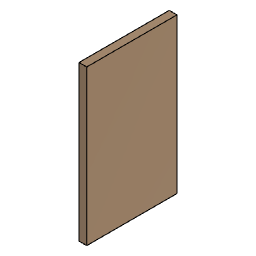
Connection box side panel (Autodesk Fusion 360 design; units mm, degrees)
Autodesk Fusion 360 part; units mm, degrees
sketch "Sketch1" plane through (0, 0, 0) normal (1, 0, 0) x (0, 1, 0)
  line L0 (35, 60) -> (-35, 60)
  line L1 (-35, 60) -> (-35, -60)
  line L2 (-35, -60) -> (35, -60)
  line L3 (35, -60) -> (35, 60)
  line L4 (35, 60) -> (-35, -60) construction
  line L5 (-35, 60) -> (35, -60) construction
  dimension "d1" = 70
  dimension "d2" = 120
  constraint perpendicular L0 L1
  constraint parallel L0 L2
  constraint parallel L1 L3
  constraint horizontal L0
  constraint coincident L4 origin
  constraint coincident L5 origin
  measures "d1" distance of L1.end L2.end
  measures "d2" distance of L0.end L1.end
extrude "Extrude1" add sketch "Sketch1" along normal blind 6
named bodies: "Panel"
